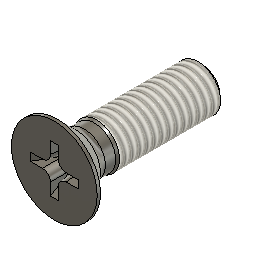
AssemblageDMXEasy (Autodesk Fusion 360 archive; units mm, degrees)
design "Vis à tête fraisée PN-EN ISO 7046-2 - M5 x 16 - H Acier 4.6 Standard"
description: Vis à tête fraisée PN-EN ISO 7046-2 - M5 x 16 - H
part number: PN-EN ISO 7046-2 - M5x16 - H Acier 4.6 Standard
Autodesk Fusion 360 part; units mm, degrees
sketch "Sketch1" plane through (0, 0, 0) normal (0, 1, 0) x (1, 0, 0)
  line L0 (0, -5) -> (-4.65, -5)
  line L1 (-4.65, -5) -> (-4.65, -4.65)
  line L2 (-4.65, -4.65) -> (-2.3, -2.3)
  line L3 (-2.5, -0.3) -> (-2.5, 11)
  line L4 (-2.5, 11) -> (0, 11)
  line L5 (0, 11) -> (0, -5)
  line L6 (-2.3, -0.6464) -> (-2.3, -2.3)
  line L7 (-2.5, -0.3) -> (-2.3, -0.6464)
  dimension "d9" = 5
  dimension "d11" = 9.3
  dimension "d71" = 2.7
  dimension "d72" = 4.6
  dimension "d89" = 11.3
  dimension "d101" = 30
  dimension "d115" = 16
  dimension "d121" = 45
  constraint perpendicular L0 L1
  constraint vertical L3
  constraint perpendicular L3 L4
  constraint perpendicular L0 L5
  constraint collinear origin L0.start L4.end
  constraint horizontal L0
  constraint coincident L2.end L6.end
  constraint coincident L6 L7.end
  constraint coincident L6.start L7.end
  constraint coincident origin L2
  measures "d71" distance of L0 L2.end
  measures "d89" distance of L4 L3.start
  measures "d101" angle of L3 L7
  measures "d115" distance of L0.start L4
  measures "d121" angle of L2 L5
revolve "Revolve1" add sketch "Sketch1" angle 360 about axis through (0, 0, -11) along (0, 0, 1) makes body 1
sketch "Sketch2" plane through (0, 0, 5) normal (0, 0, 1) x (1, 0, 0)
  line L0 (-0.4333, 0.4333) -> (-2.6, 0.4333)
  line L1 (-2.6, 0.4333) -> (-2.6, -0.4333)
  line L2 (-2.6, -0.4333) -> (-0.4333, -0.4333)
  line L3 (0.4333, -2.6) -> (0.4333, -0.4333)
  line L4 (-0.4333, -2.6) -> (0.4333, -2.6)
  line L5 (-0.4333, -0.4333) -> (-0.4333, -2.6)
  line L6 (2.6, 0.4333) -> (0.4333, 0.4333)
  line L7 (2.6, -0.4333) -> (2.6, 0.4333)
  line L8 (0.4333, -0.4333) -> (2.6, -0.4333)
  line L9 (-0.4333, 2.6) -> (-0.4333, 0.4333)
  line L10 (0.4333, 2.6) -> (-0.4333, 2.6)
  line L11 (0.4333, 0.4333) -> (0.4333, 2.6)
  dimension "d111" = 360
  dimension "d117" = 5.2
  dimension "d122" = 0.8667
  constraint horizontal L0
  constraint perpendicular L0 L1
  constraint vertical L0.start L2.end
  constraint coincident L0.start L9.end
  measures "d117" distance of L4.start L10
  measures "d122" distance of L0 L2
extrude "Extrude1" add sketch "Sketch2" against normal blind 3.2 draft -4 separate body makes body 2
draft "Draft1" angle -30 neutral plane through (0, 0, 5) pull (0, 0, 1) 4 faces at (2.5254, -0.0699, 3.9333) (0.0699, 2.5254, 3.9333) (-2.5254, -0.0699, 3.9333) (0.0699, -2.5254, 3.9333) on bodies 2
fillet "Fillet3" radius 0.8667 4 edges at (0.3215, 0.3215, 3.4) (0.3215, -0.3215, 3.4) (-0.3215, -0.3215, 3.4) (-0.3215, 0.3215, 3.4) on bodies 2
combine "Combine1" operation cut target body 1 tool bodies 2
thread "Thread1" "ISO Metric profile 5.0 M5x0.8 M5x0.8 6g" major diameter 4.901 minor diameter 3.9895 pitch 0.8 angle 60 resizes the face on face at (-2.4969, 0.1246, -3.4667) on bodies 1
fillet "Fillet5" radius 1.3 1 edges at (-2.1444, 0.8317, 2.3) on bodies 1
sketch "Sketch6" plane through (0, 0, 0) normal (0, 1, 0) x (1, 0, 0)
  line L0 (-2, 11) -> (-2.55, 11)
  line L1 (-2.55, 11) -> (-2.55, 10.5)
  line L2 (-2.55, 10.5) -> (-2, 11)
  line L3 (-2.5, 11) -> (0, 11)
  line L4 (0, 0) -> (0, 11) construction
  dimension "d102" = 2.55
  dimension "d118" = 2
  dimension "d119" = 0.5
  constraint horizontal L0
  constraint perpendicular L0 L1
  constraint coincident L0.start L3
  constraint coincident L4.start origin
  constraint coincident L3.end L4.end
  measures "d102" distance of L4.start L1
  measures "d118" distance of L0.start L4
  measures "d119" distance of L0 L1.end
revolve "Revolve3" cut sketch "Sketch6" angle 360 about axis through (0, 0, 1.75) along (0, 0, 1) bodies 1
equation "d9 = adsk_nomdia"
equation "d11 = adsk_headdia"
equation "adsk_nomlen = 16.00 mm"
equation "adsk_headh = 2.70 mm"
equation "adsk_headdia = 9.30 mm"
equation "adsk_nomdia = 5.00 mm"
equation "adsk_headang = 90.00 deg"
equation "adsk_phildia = 5.20 mm"
equation "d31 = -adsk_phildepth"
equation "adsk_philwidth = adsk_phildia / 6"
equation "adsk_phildepth = 3.20 mm"
equation "d71 = adsk_headh"
equation "d72 = adsk_shnkdia"
equation "adsk_shnkdia = adsk_nomdia - 0.5 * adsk_pitch1"
equation "d89 = adsk_thrlen"
equation "adsk_thrlen = 11.30 mm"
equation "adsk_pitch1 = 0.80 mm"
equation "adsk_startlen = adsk_nomdia * 0.1"
equation "adsk_midfillet = 1.30 mm"
equation "d96 = adsk_midfillet"
equation "d99 = ( adsk_shnkdia / 2 ) * tan(90 deg - adsk_headang / 2) + adsk_headh"
equation "d102 = adsk_nomdia * 0.51"
equation "adsk_endpointdia = adsk_nomdia - adsk_startlen * 2"
equation "d114 = adsk_philwidth"
equation "d115 = adsk_nomlen"
equation "d117 = adsk_phildia"
equation "d118 = adsk_endpointdia / 2"
equation "d119 = adsk_startlen"
equation "d121 = adsk_headang * 0.5"
equation "d122 = adsk_philwidth"

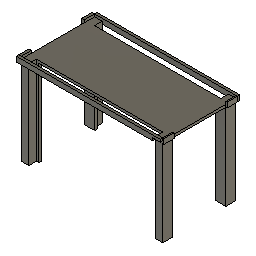
design "ESP_block_DMXEasy"
Autodesk Fusion 360 part; units mm, degrees
sketch "Esquisse1" plane through (0, 0, 0) normal (0, 0, 1) x (1, 0, 0)
  line L0 (0, 0) -> (56, 0)
  line L1 (56, 0) -> (56, 29)
  line L2 (56, 29) -> (0, 29)
  line L3 (0, 29) -> (0, 0)
  dimension "d1" = 56
  dimension "d2" = 29
  constraint horizontal L0
  constraint vertical L1
  constraint horizontal L2
  constraint vertical L3
  constraint coincident L0.start L3.end
  measures "d1" distance of L0.start L0.end
  measures "d2" distance of L0.end L1.end
extrude "Extrusion1" add sketch "Esquisse1" along normal blind 35 makes body 1
sketch "Esquisse2" plane through (0, 0, 0) normal (0, 0, -1) x (1, 0, 0)
  line L0 (0, 0) -> (0, -29)
  line L1 (0, -29) -> (56, -29)
  line L2 (56, -29) -> (56, 0)
  line L3 (56, 0) -> (0, 0)
  line L4 (56, -25) -> (0, -25)
  line L5 (0, -25) -> (0, -4)
  line L6 (0, -4) -> (56, -4)
  line L7 (56, -4) -> (56, -25)
  line L8 (52, -29) -> (4, -29)
  line L9 (4, -29) -> (4, 0)
  line L10 (4, 0) -> (52, 0)
  line L11 (52, 0) -> (52, -29)
  dimension "d5" = 4
  dimension "d6" = 4
  dimension "d7" = 4
  dimension "d8" = 4
  constraint horizontal L4
  constraint vertical L5
  constraint horizontal L6
  constraint vertical L7
  constraint coincident L0 L5.end
  constraint coincident L2 L4.start
  constraint horizontal L8
  constraint vertical L9
  constraint horizontal L10
  constraint vertical L11
  constraint coincident L3 L9.end
  constraint coincident L1 L8.start
  measures "d5" distance of L1 L4
  measures "d6" distance of L3 L6
  measures "d7" distance of L0 L9
  measures "d8" distance of L2 L11
extrude "Extrusion2" cut sketch "Esquisse2" against normal blind 34 contours L0 L4 L5 L6 L9 | L3 L6 L9 L10 L11 | L4 L6 L9 L11 | L1 L4 L8 L9 L11 | L2 L4 L6 L7 L11 bodies 1
sketch "Esquisse3" plane through (56, 0, 0) normal (1, 0, 0) x (0, 1, 0)
  line L0 (25, 34) -> (25, 0)
  line L1 (25, 0) -> (29, 0)
  line L2 (29, 0) -> (29, 35)
  line L3 (29, 35) -> (0, 35)
  line L4 (0, 35) -> (0, 0)
  line L5 (0, 0) -> (4, 0)
  line L6 (4, 0) -> (4, 34)
  line L7 (4, 34) -> (25, 34)
  line L8 (4, 35) -> (0, 35)
  line L9 (0, 35) -> (0, 34)
  line L10 (0, 34) -> (4, 34)
  line L11 (4, 34) -> (4, 35)
  line L12 (25, 34) -> (29, 34)
  line L13 (29, 34) -> (29, 35)
  line L14 (29, 35) -> (25, 35)
  line L15 (25, 35) -> (25, 34)
  dimension "d11" = 1
  dimension "d12" = 4
  constraint horizontal L8
  constraint vertical L9
  constraint horizontal L10
  constraint vertical L11
  constraint coincident L4 L9.end
  constraint coincident L3 L8.start
  constraint horizontal L12
  constraint vertical L13
  constraint horizontal L14
  constraint vertical L15
  constraint coincident L2.end L3.start
  constraint coincident L0.start L7.end
  measures "d11" distance of L8.start L6.end
  measures "d12" distance of L9.end L6.end
extrude "Extrusion3" add sketch "Esquisse3" along normal blind 0.5 contours L2 L3 L12 L13 L14 L15 | L3 L4 L8 L9 L10 L11 bodies 1
sketch "Esquisse4" plane through (0, 0, 35) normal (0, 0, 1) x (-1, 0, 0)
  line L0 (0, -29) -> (0, 0)
  line L1 (0, 0) -> (-56.5, 0)
  line L2 (-56.5, 0) -> (-56.5, -4)
  line L3 (-56.5, -4) -> (-56, -4)
  line L4 (-56, -4) -> (-56, -25)
  line L5 (-56, -25) -> (-56.5, -25)
  line L6 (-56.5, -25) -> (-56.5, -29)
  line L7 (-56.5, -29) -> (0, -29)
  line L8 (-56, -25) -> (-56.5, -25)
  line L9 (-56.5, -25) -> (-56.5, -29)
  line L10 (-56.5, -29) -> (-56, -29)
  line L11 (-56, -29) -> (-56, -25)
  line L12 (-56, 0) -> (-56.5, 0)
  line L13 (-56.5, 0) -> (-56.5, -4)
  line L14 (-56.5, -4) -> (-56, -4)
  line L15 (-56, -4) -> (-56, 0)
  dimension "d15" = 0.5
  constraint horizontal L8
  constraint vertical L9
  constraint horizontal L10
  constraint vertical L11
  constraint coincident L6.end L7.start
  constraint coincident L4.end L5.start
  constraint horizontal L12
  constraint vertical L13
  constraint horizontal L14
  constraint vertical L15
  constraint coincident L2.end L3.start
  constraint coincident L1 L12.start
  measures "d15" distance of L12.start L1.end
extrude "Extrusion4" add sketch "Esquisse4" along normal blind 1 contours L5 L6 L7 L8 L9 L10 L11 | L1 L2 L3 L12 L13 L14 L15 bodies 1
sketch "Esquisse5" plane through (0, 0, 0) normal (-1, 0, 0) x (0, -1, 0)
  line L0 (-25, 0) -> (-25, 34)
  line L1 (-25, 34) -> (-4, 34)
  line L2 (-4, 34) -> (-4, 0)
  line L3 (-4, 0) -> (0, 0)
  line L4 (0, 0) -> (0, 35)
  line L5 (0, 35) -> (-29, 35)
  line L6 (-29, 35) -> (-29, 0)
  line L7 (-29, 0) -> (-25, 0)
  line L8 (-29, 34) -> (-25, 34)
  line L9 (-25, 34) -> (-25, 35)
  line L10 (-25, 35) -> (-29, 35)
  line L11 (-29, 35) -> (-29, 34)
  line L12 (0, 35) -> (-4, 35)
  line L13 (-4, 35) -> (-4, 34)
  line L14 (-4, 34) -> (0, 34)
  line L15 (0, 34) -> (0, 35)
  dimension "d18" = 1
  dimension "d19" = 4
  constraint horizontal L8
  constraint vertical L9
  constraint horizontal L10
  constraint vertical L11
  constraint coincident L5 L9.end
  constraint coincident L6 L8.start
  constraint horizontal L12
  constraint vertical L13
  constraint horizontal L14
  constraint vertical L15
  constraint coincident L1.end L2.start
  constraint coincident L4.end L5.start
  measures "d18" distance of L8.start L5.end
  measures "d19" distance of L9.end L5.end
extrude "Extrusion5" add sketch "Esquisse5" along normal blind 1 contours L5 L6 L8 L9 L10 L11 | L4 L5 L12 L13 L14 L15 bodies 1
sketch "Esquisse6" plane through (0, 0, 35) normal (0, 0, 1) x (-1, 0, 0)
  line L0 (-56, 0) -> (-56, -4)
  line L1 (-56, -4) -> (-56, -25)
  line L2 (-56, -25) -> (-56, -29)
  line L3 (-56, -29) -> (1, -29)
  line L4 (1, -29) -> (1, -25)
  line L5 (1, -25) -> (0, -25)
  line L6 (0, -25) -> (0, -4)
  line L7 (0, -4) -> (1, -4)
  line L8 (1, -4) -> (1, 0)
  line L9 (1, 0) -> (-56, 0)
  line L10 (0, -4) -> (1, -4)
  line L11 (1, -4) -> (1, 0)
  line L12 (1, 0) -> (0, 0)
  line L13 (0, 0) -> (0, -4)
  line L14 (0, -29) -> (1, -29)
  line L15 (1, -29) -> (1, -25)
  line L16 (1, -25) -> (0, -25)
  line L17 (0, -25) -> (0, -29)
  dimension "d22" = 1
  constraint horizontal L10
  constraint vertical L11
  constraint horizontal L12
  constraint vertical L13
  constraint coincident L8.end L9.start
  constraint coincident L6.end L7.start
  constraint horizontal L14
  constraint vertical L15
  constraint horizontal L16
  constraint vertical L17
  constraint coincident L4.end L5.start
  measures "d22" distance of L4.end L5.end
extrude "Extrusion6" add sketch "Esquisse6" along normal blind 1 contours L7 L8 L9 L10 L11 L12 L13 | L3 L4 L5 L14 L15 L16 L17 bodies 1
sketch "Esquisse7" plane through (0, 0, 35) normal (0, 0, 1) x (-1, 0, 0)
  line L0 (0, -29) -> (0, -25)
  line L1 (0, -25) -> (0, -4)
  line L2 (0, -4) -> (0, 0)
  line L3 (0, 0) -> (-56, 0)
  line L4 (-56, 0) -> (-56, -4)
  line L5 (-56, -4) -> (-56, -25)
  line L6 (-56, -25) -> (-56, -29)
  line L7 (-56, -29) -> (0, -29)
  line L8 (-3, -29) -> (-53, -29)
  line L9 (-53, -29) -> (-53, -26)
  line L10 (-53, -26) -> (-3, -26)
  line L11 (-3, -26) -> (-3, -29)
  line L12 (-53, 0) -> (-3, 0)
  line L13 (-3, 0) -> (-3, -3)
  line L14 (-3, -3) -> (-53, -3)
  line L15 (-53, -3) -> (-53, 0)
  dimension "d25" = 3
  dimension "d26" = 3
  dimension "d27" = 3
  dimension "d28" = 3
  dimension "d29" = 3
  dimension "d30" = 3
  constraint horizontal L8
  constraint vertical L9
  constraint horizontal L10
  constraint vertical L11
  constraint coincident L7 L8.start
  constraint horizontal L12
  constraint vertical L13
  constraint horizontal L14
  constraint vertical L15
  constraint coincident L3 L12.start
  measures "d25" distance of L0 L11
  measures "d26" distance of L6 L9
  measures "d27" distance of L8.end L9.end
  measures "d28" distance of L2 L13
  measures "d29" distance of L4 L15
  measures "d30" distance of L12.start L14.end
extrude "Extrusion7" cut sketch "Esquisse7" against normal through all contours L7 L8 L9 L10 L11 | L3 L12 L13 L14 L15 bodies 1
sketch "Esquisse8" plane through (0, 0, 0) normal (0, -1, 0) x (1, 0, 0)
  line L0 (53, 35) -> (53, 0)
  line L1 (53, 0) -> (56, 0)
  line L2 (56, 0) -> (56, 34)
  line L3 (56, 34) -> (56.5, 34)
  line L4 (56.5, 34) -> (56.5, 36)
  line L5 (56.5, 36) -> (56, 36)
  line L6 (56, 36) -> (56, 35)
  line L7 (56, 35) -> (53, 35)
  line L8 (56.5, 34) -> (-1, 34)
  line L9 (-1, 34) -> (-1, 36)
  line L10 (-1, 36) -> (56.5, 36)
  line L11 (56.5, 36) -> (56.5, 34)
  dimension "d38" = 2
  dimension "d39" = 57.5
  constraint horizontal L8
  constraint vertical L9
  constraint horizontal L10
  constraint vertical L11
  constraint coincident L3.end L4.start
  measures "d38" distance of L3.end L4.end
  measures "d39" distance of L9.end L4.end
extrude "Extrusion8" add sketch "Esquisse8" along normal blind 1 separate body contours L0 L6 L7 L8 L9 L10 makes body 2
sketch "Esquisse9" plane through (0, 29, 0) normal (0, 1, 0) x (-1, 0, 0)
  line L0 (-3, 35) -> (-3, 0)
  line L1 (-3, 0) -> (0, 0)
  line L2 (0, 0) -> (0, 34)
  line L3 (0, 34) -> (1, 34)
  line L4 (1, 34) -> (1, 36)
  line L5 (1, 36) -> (0, 36)
  line L6 (0, 36) -> (0, 35)
  line L7 (0, 35) -> (-3, 35)
  line L8 (1, 34) -> (-56.5, 34)
  line L9 (-56.5, 34) -> (-56.5, 36)
  line L10 (-56.5, 36) -> (1, 36)
  line L11 (1, 36) -> (1, 34)
  dimension "d34" = 2
  dimension "d35" = 57.5
  constraint horizontal L8
  constraint vertical L9
  constraint horizontal L10
  constraint vertical L11
  constraint coincident L3.end L4.start
  measures "d34" distance of L3.end L4.end
  measures "d35" distance of L3.end L8.end
extrude "Extrusion9" add sketch "Esquisse9" along normal blind 1 separate body contours L0 L6 L7 L8 L9 L10 makes body 3

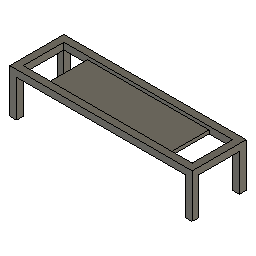
design "MAX485_DMXEasy"
Autodesk Fusion 360 part; units mm, degrees
sketch "Esquisse1" plane through (0, 0, 0) normal (0, 0, 1) x (1, 0, 0)
  line L0 (0, 0) -> (54, 0)
  line L1 (54, 0) -> (54, 16)
  line L2 (54, 16) -> (0, 16)
  line L3 (0, 16) -> (0, 0)
  dimension "d1" = 16
  dimension "d2" = 54
  constraint horizontal L0
  constraint vertical L1
  constraint horizontal L2
  constraint vertical L3
  constraint coincident L0.start L3.end
  measures "d1" distance of L0.start L2.end
  measures "d2" distance of L1.end L2.end
extrude "Extrusion1" add sketch "Esquisse1" along normal blind 13
sketch "Esquisse2" plane through (0, 0, 13) normal (0, 0, 1) x (-1, 0, 0)
  line L0 (0, -16) -> (0, 0)
  line L1 (0, 0) -> (-54, 0)
  line L2 (-54, 0) -> (-54, -16)
  line L3 (-54, -16) -> (0, -16)
  line L4 (-2, -14) -> (-52, -14)
  line L5 (-52, -14) -> (-52, -2)
  line L6 (-52, -2) -> (-2, -2)
  line L7 (-2, -2) -> (-2, -14)
  dimension "d5" = 2
  dimension "d6" = 2
  dimension "d7" = 2
  dimension "d8" = 2
  constraint horizontal L4
  constraint vertical L5
  constraint horizontal L6
  constraint vertical L7
  measures "d5" distance of L3 L4
  measures "d6" distance of L2 L5
  measures "d7" distance of L1 L6
  measures "d8" distance of L0 L7
extrude "Extrusion2" cut sketch "Esquisse2" against normal blind 1 contours L4 L5 L6 L7
extrude "Extrusion3" cut 1 faces at (35.3333, 10, 12) along direction (0, 0, -1) blind 10 from surface at 2
sketch "Esquisse3" plane through (0, 0, 0) normal (0, -1, 0) x (1, 0, 0)
  line L0 (0, 0) -> (54, 0)
  line L1 (54, 0) -> (54, 13)
  line L2 (54, 13) -> (0, 13)
  line L3 (0, 13) -> (0, 0)
  line L4 (2, 0) -> (52, 0)
  line L5 (52, 0) -> (52, 11)
  line L6 (52, 11) -> (2, 11)
  line L7 (2, 11) -> (2, 0)
  dimension "d14" = 2
  dimension "d15" = 2
  dimension "d16" = 2
  constraint horizontal L4
  constraint vertical L5
  constraint horizontal L6
  constraint vertical L7
  constraint coincident L0 L4.start
  measures "d14" distance of L3 L7
  measures "d15" distance of L2 L6
  measures "d16" distance of L1 L5
extrude "Extrusion4" cut sketch "Esquisse3" against normal blind 16 contours L0 L4 L5 L6 L7
sketch "Esquisse4" plane through (54, 0, 0) normal (1, 0, 0) x (0, 1, 0)
  line L0 (0, 0) -> (16, 0)
  line L1 (16, 0) -> (16, 13)
  line L2 (16, 13) -> (0, 13)
  line L3 (0, 13) -> (0, 0)
  line L4 (2, 0) -> (14, 0)
  line L5 (14, 0) -> (14, 11)
  line L6 (14, 11) -> (2, 11)
  line L7 (2, 11) -> (2, 0)
  dimension "d19" = 2
  dimension "d20" = 2
  dimension "d21" = 2
  constraint horizontal L4
  constraint vertical L5
  constraint horizontal L6
  constraint vertical L7
  constraint coincident L0 L4.start
  measures "d19" distance of L3 L7
  measures "d20" distance of L1 L5
  measures "d21" distance of L2 L6
extrude "Extrusion5" cut sketch "Esquisse4" against normal through all contours L0 L4 L5 L6 L7
sketch "Esquisse5" plane through (0, 0, 12) normal (0, 0, 1) x (-1, 0, 0)
  line L0 (-2, -2) -> (-52, -2)
  line L1 (-52, -2) -> (-52, -14)
  line L2 (-52, -14) -> (-2, -14)
  line L3 (-2, -14) -> (-2, -2)
  line L4 (-52, -14) -> (-45, -14)
  line L5 (-45, -14) -> (-45, -2)
  line L6 (-45, -2) -> (-52, -2)
  line L7 (-52, -2) -> (-52, -14)
  line L8 (-2, -14) -> (-9, -14)
  line L9 (-9, -14) -> (-9, -2)
  line L10 (-9, -2) -> (-2, -2)
  line L11 (-2, -2) -> (-2, -14)
  dimension "d23" = 7
  dimension "d24" = 7
  constraint horizontal L4
  constraint vertical L5
  constraint horizontal L6
  constraint vertical L7
  constraint coincident L0 L5.end
  constraint coincident L1.end L2.start
  constraint horizontal L8
  constraint vertical L9
  constraint horizontal L10
  constraint vertical L11
  constraint coincident L0 L9.end
  constraint coincident L2.end L3.start
  measures "d23" distance of L2.end L8.end
  measures "d24" distance of L1.end L4.end
extrude "Extrusion6" cut sketch "Esquisse5" against normal through all contours L0 L2 L3 L8 L9 L10 L11 | L0 L1 L2 L4 L5 L6 L7
